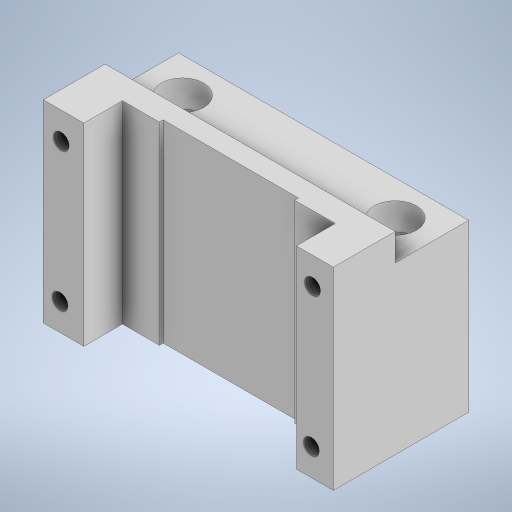
# Autodesk Inventor part: Lose Backe
Saved by Autodesk Inventor 2023 (Build 270158000, 158)
## iProperties
Created: 2023-05-10
Part Number: Lose Backe
Material: Generic
Document SubType Name: Modeling
Designer: dell
Density: 1 g/cm^3
Appearance: Default
Author: dell
Autodesk Inventor part; units mm, degrees
ref_plane "YZ Plane" through (0, 0, 0) normal (1, 0, 0) x (0, 1, 0)
ref_plane "XZ Plane" through (0, 0, 0) normal (0, 1, 0) x (-1, 0, 0)
ref_plane "XY Plane" through (0, 0, 0) normal (0, 0, 1) x (1, 0, 0)
sketch "Sketch1" plane through (0, 0, 0) normal (1, 0, 0) x (0, 1, 0)
  line L0 (-21.5, -17.5) -> (21.5, -17.5)
  line L1 (21.5, -17.5) -> (21.5, 1.5)
  line L2 (21.5, 17.5) -> (-21.5, 17.5)
  line L3 (-21.5, 17.5) -> (-21.5, -17.5)
  line L4 (-21.5, -17.5) -> (21.5, 17.5) construction
  line L5 (21.5, -17.5) -> (-21.5, 17.5) construction
  line L6 (18.0188, 17.5) -> (28.5, 17.5)
  line L7 (28.5, 17.5) -> (28.5, 1.5)
  line L8 (28.5, 1.5) -> (21.5, 1.5)
  point P0 (0, 0)
  dimension "d0" = 43
  dimension "d1" = 35
  dimension "d2" = 50
  dimension "d3" = 16
  constraints: 18 end point, 3 perpendicular, 2 horizontal, 2 midpoint, 2 parallel
  measures "d0" distance of L0.start L0.end
  measures "d1" distance of L0.end L2.start
  measures "d2" distance of L2.end L6.end
  measures "d3" distance of L6.end L7.end
extrude "Extrusion1" add sketch "Sketch1" along normal blind 75
sketch "Sketch2" plane through (0, 28.5, 17.5) normal (0, 1, 0) x (1, 0, 0)
  line L0 (0, 0) -> (75, 0) projected
  line L1 (65.4712, 0) -> (65.4712, 10)
  line L2 (65.4712, 10) -> (55, 10)
  line L3 (55, 10) -> (55, 11)
  line L4 (55, 11) -> (20, 11)
  line L5 (20, 11) -> (20, 10)
  line L6 (20, 10) -> (10.4712, 10)
  line L7 (10.4712, 10) -> (10.4712, 0)
  line L8 (0, 35) -> (75, 35) projected
  line L9 (37.5, 35) -> (37.5, 5.3668)
  point P0 (0, 17.5)
  dimension "d6" = 55
  dimension "d7" = 35
  dimension "d8" = 17.5
  dimension "d9" = 11
  dimension "d10" = 10
  constraints: 16 end point, 4 perpendicular, 4 point on line, 2 vertical, 1 horizontal, 1 midpoint
  measures "d6" distance between parallel lines of L7 L1
  measures "d7" distance between parallel lines of L5 L3
  measures "d8" distance between parallel lines of L5 L9
  measures "d9" distance between parallel lines of L0 L4
  measures "d10" distance between parallel lines of L0 L2
extrude "Extrusion2" cut sketch "Sketch2" against normal blind 75
sketch "Sketch3" plane through (0, 21.5, 1.5) normal (0, 1, 0) x (1, 0, 0)
  circle A0 centre (10, 10) radius 5.5
  circle A1 centre (65, 10) radius 5.5
  line L0 (0, 19) -> (75, 19) projected
  line L1 (75, 19) -> (75, 0) projected
  line L2 (0, -16) -> (10.4712, -16) projected
  line L3 (65.4712, -16) -> (75, -16) projected
  point P0 (0, 1.5)
  dimension "d13" = 11
  dimension "d14" = 11
  dimension "d15" = 55
  dimension "d19" = 26
  dimension "d20" = 26
  constraints: 2 centre point
  measures "d13" diameter of A1
  measures "d14" diameter of A0
  measures "d15" distance of A1.centre A0.centre
  measures "d19" distance from line of L2 A0.centre
  measures "d20" distance from line of L3 A1.centre
extrude "Extrusion3" cut sketch "Sketch3" against normal blind 7
sketch "Sketch4" plane through (65, 14.5, -8.5) normal (0, 1, 0) x (1, 0, 0)
  circle A0 centre (0, 0) radius 5.5 projected
  circle A1 centre (0, 0) radius 3.2
  circle A2 centre (-55, 0) radius 5.5 projected
  circle A3 centre (-55, 0) radius 3.2
  point P0 (-65, -8.5)
  dimension "d23" = 6.4
  dimension "d24" = 6.4
  constraints: 2 centre point, 2 coincident
  measures "d23" diameter of A3
  measures "d24" diameter of A1
extrude "Extrusion4" cut sketch "Sketch4" against normal blind 40 contours A1 | A3
sketch "Sketch7" plane through (0, -21.5, 17.5) normal (0, 0, 1) x (1, 0, 0)
  line L0 (0, 0) -> (10.4712, 0) projected
  line L1 (0, 50) -> (10.4712, 50) projected
  point P0 (0, 21.5)
  point P1 (4.3276, 7)
  point P2 (4.6222, 43)
  point P3 (5.2356, 0)
  dimension "d31" = 7
  dimension "d32" = 36
  dimension "d33" = 7
  constraints: 1 midpoint
  measures "d31" vertical distance of point (5.236, 0) point (4.328, 7)
  measures "d32" vertical distance of point (4.328, 7) point (4.622, 43)
  measures "d33" distance from line of L1 point (4.622, 43)
hole "Hole1" at (4.3276, -14.5, 17.5) at (4.6222, 21.5, 17.5) direction (0, 0, -1) diameter 4.134 depth 14.2 tip angle 118 thread size "M5x0.8" class "6H" standard "ISO Metric profile"
pattern_linear "Rectangular Pattern1" count 2 spacing 65 along (1, 0, 0) of "Hole1"
sketch "Sketch9" plane through (0, -21.5, -17.5) normal (0, -1, 0) x (1, 0, 0)
  circle A0 centre (37.5, 11) radius 6
  line L0 (0, 35) -> (0, 0) projected
  line L1 (0, 35) -> (10.4712, 35) projected
  point P0 (0, 17.5)
  dimension "d53" = 37.5
  dimension "d54" = 24
  dimension "d55" = 12
  constraints: 1 centre point
  measures "d53" distance from line of L0 A0.centre
  measures "d54" distance from line of L1 A0.centre
  measures "d55" diameter of A0
extrude "Extrusion6" cut sketch "Sketch9" against normal blind 20
sketch "Sketch10" plane through (0, -21.5, -17.5) normal (0, 0, -1) x (-1, 0, 0)
  line L0 (0, 0) -> (0, 43) projected
  line L1 (0, 0) -> (-75, 0) projected
  line L2 (-75, 0) -> (-75, 43) projected
  point P0 (0, 21.5)
  point P1 (-34, 7)
  dimension "d59" = 7
  dimension "d60" = 41
  measures "d59" distance from line of L1 point (-34, 7)
  measures "d60" distance from line of L2 point (-34, 7)
hole "Hole3" at (34, -14.5, -17.5) direction (0, 0, 1) diameter 2.459 depth 8.8 tip angle 118 thread size "M3x0.5" class "6H" standard "ISO Metric profile"
body "Solid1"
